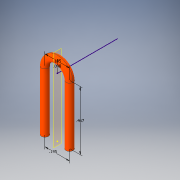
# Autodesk Inventor part: Sun_SmallStaple
Saved by Autodesk Inventor 2016 (Build 200138000, 138)
## iProperties
Created: 2017-11-13
Part Number: Sun_SmallStaple
Material: Generic
Document SubType Name: Modeling
Designer: sun01147
Density: 1 g/cm^3
Appearance: Default
Mass: 0.0482886 g
Surface Area: 1.41329 cm^2
Volume: 0.0482886 cm^3
Author: sun01147
Autodesk Inventor part; units mm, degrees
ref_plane "XZ Plane" through (0, 0, 0) normal (0, 1, 0) x (-1, 0, 0)
ref_plane "XY Plane" through (0, 0, 0) normal (0, 0, 1) x (1, 0, 0)
sketch "Sketch1" plane through (0, 0, 0) normal (0, 0, 1) x (1, 0, 0)
  line L0 (4.953, 0) -> (4.953, 11.8618)
  line L1 (0, 11.8618) -> (0, 0)
  arc A0 (4.953, 11.8618) -> (0, 11.8618) centre (2.4765, 11.8618) ccw
  dimension "d0" = 4.953
  dimension "d1" = 11.8618
  dimension "d2" = 2.4765
  dimension "d3" = 4.953
  constraints: 4 end point, 2 parallel, 2 point on circle, 1 centre point, 1 vertical
  measures "d0" distance of L1.start L0.end
  measures "d1" distance of L0.end L0.start
  measures "d2" radius of A0
  measures "d3" distance between parallel lines of L1 L0
sketch "Sketch6" plane through (0, 0, 0) normal (0, 1, 0) x (-1, 0, 0)
  circle A0 centre (0, 0) radius 0.6985
  dimension "d4" = 1.397
  constraints: 1 centre point, 1 coincident
  measures "d4" diameter of A0
sweep "Sweep1" add profiles "Sketch6" path "Sketch1"
ref_plane "Work Plane1" through (2.4765, 11.8618, 0) normal (1, 0, 0) x (0, 1, 0)
sketch "Sketch8" plane through (2.4765, 11.8618, 0) normal (1, 0, 0) x (0, 1, 0)
  line L0 (0, 0) -> (0, -12.0654)
  point P0 (-11.8618, 0)
  constraints: 2 end point, 2 vertical
body "Solid1"
